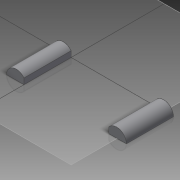
# Autodesk Inventor part: Bad PillarS
Saved by Autodesk Inventor 2018 (Build 220112000, 112)
## iProperties
Created: 2017-12-11
Part Number: Bad PillarS
Material: Generic
Document SubType Name: Modeling
Designer: Rus
Density: 1 g/cm^3
Appearance: Default
Author: Rus
Autodesk Inventor part; units mm, degrees
ref_plane "YZ Plane" through (0, 0, 0) normal (1, 0, 0) x (0, 1, 0)
ref_plane "XZ Plane" through (0, 0, 0) normal (0, 1, 0) x (-1, 0, 0)
sketch "Sketch1" plane through (0, 0, 0) normal (0, 0, 1) x (1, 0, 0)
  arc A0 (0, 6.35) -> (-19.1337, 0) centre (-8.4667, -0.1401) ccw projected
  line L0 (0, 0) -> (-19.1337, 0) projected
  line L1 (0, 6.35) -> (0, 0) projected
  line L2 (92.6375, 6.35) -> (92.6375, 0) projected
  line L3 (92.6375, 0) -> (111.7712, 0) projected
  arc A1 (111.7712, 0) -> (92.6375, 6.35) centre (101.1041, -0.1401) ccw projected
ref_plane "Work Plane1" through (-19.1337, 0, 51.4547) normal (0, 0, -1) x (0, 1, 0)
extrude "Extrusion1" add sketch "Sketch1" along normal up to surface (51.4547 mm away)
body "Solid1"
